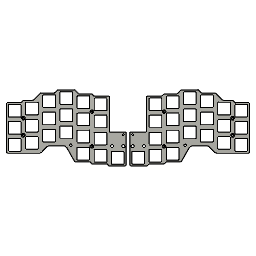
mriya-cnc-top-plate-v.1.01 (Autodesk Fusion 360 design; units mm, degrees)
Autodesk Fusion 360 part; units mm, degrees
sketch "mriya-top-plate" plane through (0, 0, 0) normal (0, 0, 1) x (1, 0, 0)
  line L0 (-96.0213, 15.6719) -> (-89.7787, 21.9145) construction
  line L1 (-21.4858, 1.079) -> (-22.6142, 2.2074) construction
  line L2 (-133.1, 14.7932) -> (-98.1426, 14.7932) construction
  line L3 (-39.0716, 2.7932) -> (-24.0284, 2.7932) construction
  line L4 (-3.6, 0.4932) -> (-20.0716, 0.4932) construction
  line L5 (-59.4741, 6.1094) -> (-67.7517, 20.7608) construction
  line L6 (-40.4858, 3.379) -> (-41.6142, 4.5074) construction
  line L7 (-117.6142, 71.579) -> (-116.4858, 72.7074) construction
  line L8 (-96.0716, 81.2932) -> (-82.2284, 81.2932) construction
  line L9 (-133.1, 70.9932) -> (-119.0284, 70.9932) construction
  line L10 (-87.6574, 22.7932) -> (-71.2344, 22.7932) construction
  line L11 (-43.0284, 5.0932) -> (-57.7328, 5.0932) construction
  line L12 (-77.0716, 84.7932) -> (-59.7284, 84.7932) construction
  line L13 (-53.5716, 80.2932) -> (-40.7284, 80.2932) construction
  line L14 (-20.6, 20.2932) -> (-20.6, 77.9932) construction
  line L15 (-78.4858, 84.2074) -> (-80.8142, 81.879) construction
  line L16 (-58.3142, 84.2074) -> (-54.9858, 80.879) construction
  line L17 (-134.6, 69.4932) -> (-134.6, 16.2932) construction
  line L18 (-38.1858, 78.579) -> (-39.3142, 79.7074) construction
  line L19 (-94.4, 40.3932) -> (-94.4, 27.9932)
  line L20 (-93.6, 41.1932) -> (-81.2, 41.1932)
  line L21 (-93.6, 27.1932) -> (-81.2, 27.1932)
  line L22 (-80.4, 40.3932) -> (-80.4, 27.9932)
  line L23 (-37.4, 56.0932) -> (-37.4, 43.6932)
  line L24 (-36.6, 56.8932) -> (-24.2, 56.8932)
  line L25 (-36.6, 42.8932) -> (-24.2, 42.8932)
  line L26 (-23.4, 56.0932) -> (-23.4, 43.6932)
  line L27 (-56.4, 58.3932) -> (-56.4, 45.9932)
  line L28 (-55.6, 59.1932) -> (-43.2, 59.1932)
  line L29 (-55.6, 45.1932) -> (-43.2, 45.1932)
  line L30 (-42.4, 58.3932) -> (-42.4, 45.9932)
  line L31 (-132.4, 68.0932) -> (-132.4, 55.6932)
  line L32 (-131.6, 68.8932) -> (-119.2, 68.8932)
  line L33 (-131.6, 54.8932) -> (-119.2, 54.8932)
  line L34 (-118.4, 68.0932) -> (-118.4, 55.6932)
  line L35 (-56.4, 39.3932) -> (-56.4, 26.9932)
  line L36 (-55.6, 40.1932) -> (-43.2, 40.1932)
  line L37 (-55.6, 26.1932) -> (-43.2, 26.1932)
  line L38 (-42.4, 39.3932) -> (-42.4, 26.9932)
  line L39 (-37.4, 18.0932) -> (-37.4, 5.6932)
  line L40 (-36.6, 18.8932) -> (-24.2, 18.8932)
  line L41 (-36.6, 4.8932) -> (-24.2, 4.8932)
  line L42 (-23.4, 18.0932) -> (-23.4, 5.6932)
  line L43 (-18.4, 15.7932) -> (-18.4, 3.3932)
  line L44 (-17.6, 16.5932) -> (-5.2, 16.5932)
  line L45 (-17.6, 2.5932) -> (-5.2, 2.5932)
  line L46 (-4.4, 15.7932) -> (-4.4, 3.3932)
  line L47 (-132.4, 49.0932) -> (-132.4, 36.6932)
  line L48 (-131.6, 49.8932) -> (-119.2, 49.8932)
  line L49 (-131.6, 35.8932) -> (-119.2, 35.8932)
  line L50 (-118.4, 49.0932) -> (-118.4, 36.6932)
  line L51 (-113.4, 51.3932) -> (-113.4, 38.9932)
  line L52 (-112.6, 52.1932) -> (-100.2, 52.1932)
  line L53 (-112.6, 38.1932) -> (-100.2, 38.1932)
  line L54 (-99.4, 51.3932) -> (-99.4, 38.9932)
  line L55 (-132.4, 30.0932) -> (-132.4, 17.6932)
  line L56 (-131.6, 30.8932) -> (-119.2, 30.8932)
  line L57 (-131.6, 16.8932) -> (-119.2, 16.8932)
  line L58 (-118.4, 30.0932) -> (-118.4, 17.6932)
  line L59 (-56.4, 20.3932) -> (-56.4, 7.9932)
  line L60 (-55.6, 21.1932) -> (-43.2, 21.1932)
  line L61 (-55.6, 7.1932) -> (-43.2, 7.1932)
  line L62 (-42.4, 20.3932) -> (-42.4, 7.9932)
  line L63 (-75.4, 43.8932) -> (-75.4, 31.4932)
  line L64 (-74.6, 44.6932) -> (-62.2, 44.6932)
  line L65 (-74.6, 30.6932) -> (-62.2, 30.6932)
  line L66 (-61.4, 43.8932) -> (-61.4, 31.4932)
  line L67 (-75.4, 81.8932) -> (-75.4, 69.4932)
  line L68 (-74.6, 82.6932) -> (-62.2, 82.6932)
  line L69 (-74.6, 68.6932) -> (-62.2, 68.6932)
  line L70 (-61.4, 81.8932) -> (-61.4, 69.4932)
  line L71 (-37.4, 37.0932) -> (-37.4, 24.6932)
  line L72 (-36.6, 37.8932) -> (-24.2, 37.8932)
  line L73 (-36.6, 23.8932) -> (-24.2, 23.8932)
  line L74 (-23.4, 37.0932) -> (-23.4, 24.6932)
  line L75 (-113.4, 32.3932) -> (-113.4, 19.9932)
  line L76 (-112.6, 33.1932) -> (-100.2, 33.1932)
  line L77 (-112.6, 19.1932) -> (-100.2, 19.1932)
  line L78 (-99.4, 32.3932) -> (-99.4, 19.9932)
  line L79 (-56.4, 77.3932) -> (-56.4, 64.9932)
  line L80 (-55.6, 78.1932) -> (-43.2, 78.1932)
  line L81 (-55.6, 64.1932) -> (-43.2, 64.1932)
  line L82 (-42.4, 77.3932) -> (-42.4, 64.9932)
  line L83 (-37.4, 75.0932) -> (-37.4, 62.6932)
  line L84 (-36.6, 75.8932) -> (-24.2, 75.8932)
  line L85 (-36.6, 61.8932) -> (-24.2, 61.8932)
  line L86 (-23.4, 75.0932) -> (-23.4, 62.6932)
  line L87 (-113.4, 70.3932) -> (-113.4, 57.9932)
  line L88 (-112.6, 71.1932) -> (-100.2, 71.1932)
  line L89 (-112.6, 57.1932) -> (-100.2, 57.1932)
  line L90 (-99.4, 70.3932) -> (-99.4, 57.9932)
  line L91 (-94.4, 59.3932) -> (-94.4, 46.9932)
  line L92 (-93.6, 60.1932) -> (-81.2, 60.1932)
  line L93 (-93.6, 46.1932) -> (-81.2, 46.1932)
  line L94 (-80.4, 59.3932) -> (-80.4, 46.9932)
  line L95 (-75.4, 62.8932) -> (-75.4, 50.4932)
  line L96 (-74.6, 63.6932) -> (-62.2, 63.6932)
  line L97 (-74.6, 49.6932) -> (-62.2, 49.6932)
  line L98 (-61.4, 62.8932) -> (-61.4, 50.4932)
  line L99 (-94.4, 78.3932) -> (-94.4, 65.9932)
  line L100 (-93.6, 79.1932) -> (-81.2, 79.1932)
  line L101 (-93.6, 65.1932) -> (-81.2, 65.1932)
  line L102 (-80.4, 78.3932) -> (-80.4, 65.9932)
  circle A0 centre (-115.9, 53.5432) radius 1
  circle A1 centre (-115.9, 34.5432) radius 1
  circle A2 centre (-63.3, 23.4932) radius 1.3
  circle A3 centre (-39.9, 22.5432) radius 1
  circle A4 centre (-39.9, 60.5432) radius 1
  arc A5 (-38.1858, 78.579) -> (-36.7716, 77.9932) centre (-36.7716, 79.9932) ccw construction
  arc A6 (-39.3142, 79.7074) -> (-40.7284, 80.2932) centre (-40.7284, 78.2932) ccw construction
  arc A7 (-54.9858, 80.879) -> (-53.5716, 80.2932) centre (-53.5716, 82.2931) ccw construction
  arc A8 (-58.3142, 84.2074) -> (-59.7284, 84.7932) centre (-59.7284, 82.7932) ccw construction
  arc A9 (-77.0716, 84.7932) -> (-78.4858, 84.2074) centre (-77.0716, 82.7933) ccw construction
  arc A10 (-82.2284, 81.2932) -> (-80.8142, 81.879) centre (-82.2284, 83.2932) ccw construction
  arc A11 (-96.0716, 81.2932) -> (-97.4858, 80.7074) centre (-96.0716, 79.2933) ccw construction
  arc A12 (-115.0716, 73.2932) -> (-116.4858, 72.7074) centre (-115.0716, 71.2933) ccw construction
  arc A13 (-119.0284, 70.9932) -> (-117.6142, 71.579) centre (-119.0284, 72.9932) ccw construction
  arc A14 (-133.1, 70.9932) -> (-134.6, 69.4932) centre (-133.1, 69.4932) ccw construction
  arc A15 (-134.6, 16.2932) -> (-133.1, 14.7932) centre (-133.1, 16.2932) ccw construction
  arc A16 (-98.1426, 14.7932) -> (-96.0213, 15.6719) centre (-98.1426, 17.7931) ccw construction
  arc A17 (-87.6574, 22.7932) -> (-89.7787, 21.9145) centre (-87.6573, 19.7931) ccw construction
  arc A18 (-67.7517, 20.7608) -> (-71.2344, 22.7932) centre (-71.2344, 18.793) ccw construction
  arc A19 (-59.4741, 6.1094) -> (-57.7328, 5.0932) centre (-57.7328, 7.0932) ccw construction
  arc A20 (-41.6142, 4.5074) -> (-43.0284, 5.0932) centre (-43.0284, 3.0933) ccw construction
  arc A21 (-40.4858, 3.379) -> (-39.0716, 2.7932) centre (-39.0716, 4.7932) ccw construction
  arc A22 (-22.6142, 2.2074) -> (-24.0284, 2.7932) centre (-24.0284, 0.7933) ccw construction
  arc A23 (-21.4858, 1.079) -> (-20.0716, 0.4932) centre (-20.0716, 2.4932) ccw construction
  arc A24 (-3.6, 0.4932) -> (-2.1, 1.9932) centre (-3.6, 1.9932) ccw construction
  line L103 (-2.1, 1.9932) -> (-2.1, 76.4932) construction
  line L104 (-36.7716, 77.9932) -> (-3.6, 77.9932) construction
  arc A25 (-131.6, 68.8932) -> (-132.4, 68.0932) centre (-131.6, 68.0932) ccw
  arc A26 (-118.4, 68.0932) -> (-119.2, 68.8932) centre (-119.2, 68.0932) ccw
  arc A27 (-119.2, 54.8932) -> (-118.4, 55.6932) centre (-119.2, 55.6932) ccw
  arc A28 (-132.4, 55.6932) -> (-131.6, 54.8932) centre (-131.6, 55.6932) ccw
  arc A29 (-131.6, 49.8932) -> (-132.4, 49.0932) centre (-131.6, 49.0932) ccw
  arc A30 (-118.4, 49.0932) -> (-119.2, 49.8932) centre (-119.2, 49.0932) ccw
  arc A31 (-119.2, 35.8932) -> (-118.4, 36.6932) centre (-119.2, 36.6932) ccw
  arc A32 (-132.4, 36.6932) -> (-131.6, 35.8932) centre (-131.6, 36.6932) ccw
  arc A33 (-131.6, 30.8932) -> (-132.4, 30.0932) centre (-131.6, 30.0932) ccw
  arc A34 (-118.4, 30.0932) -> (-119.2, 30.8932) centre (-119.2, 30.0932) ccw
  arc A35 (-119.2, 16.8932) -> (-118.4, 17.6932) centre (-119.2, 17.6932) ccw
  arc A36 (-132.4, 17.6932) -> (-131.6, 16.8932) centre (-131.6, 17.6932) ccw
  arc A37 (-113.4, 19.9932) -> (-112.6, 19.1932) centre (-112.6, 19.9932) ccw
  arc A38 (-100.2, 19.1932) -> (-99.4, 19.9932) centre (-100.2, 19.9932) ccw
  arc A39 (-99.4, 32.3932) -> (-100.2, 33.1932) centre (-100.2, 32.3932) ccw
  arc A40 (-112.6, 33.1932) -> (-113.4, 32.3932) centre (-112.6, 32.3932) ccw
  arc A41 (-100.2, 38.1932) -> (-99.4, 38.9932) centre (-100.2, 38.9932) ccw
  arc A42 (-113.4, 38.9932) -> (-112.6, 38.1932) centre (-112.6, 38.9932) ccw
  arc A43 (-112.6, 52.1932) -> (-113.4, 51.3932) centre (-112.6, 51.3932) ccw
  arc A44 (-99.4, 51.3932) -> (-100.2, 52.1932) centre (-100.2, 51.3932) ccw
  arc A45 (-113.4, 57.9932) -> (-112.6, 57.1932) centre (-112.6, 57.9932) ccw
  arc A46 (-100.2, 57.1932) -> (-99.4, 57.9932) centre (-100.2, 57.9932) ccw
  arc A47 (-99.4, 70.3932) -> (-100.2, 71.1932) centre (-100.2, 70.3932) ccw
  arc A48 (-112.6, 71.1932) -> (-113.4, 70.3932) centre (-112.6, 70.3932) ccw
  arc A49 (-93.6, 79.1932) -> (-94.4, 78.3932) centre (-93.6, 78.3932) ccw
  arc A50 (-80.4, 78.3932) -> (-81.2, 79.1932) centre (-81.2, 78.3932) ccw
  arc A51 (-81.2, 65.1932) -> (-80.4, 65.9932) centre (-81.2, 65.9932) ccw
  arc A52 (-94.4, 65.9932) -> (-93.6, 65.1932) centre (-93.6, 65.9932) ccw
  arc A53 (-93.6, 60.1932) -> (-94.4, 59.3932) centre (-93.6, 59.3932) ccw
  arc A54 (-80.4, 59.3932) -> (-81.2, 60.1932) centre (-81.2, 59.3932) ccw
  arc A55 (-81.2, 46.1932) -> (-80.4, 46.9932) centre (-81.2, 46.9932) ccw
  arc A56 (-94.4, 46.9932) -> (-93.6, 46.1932) centre (-93.6, 46.9932) ccw
  arc A57 (-93.6, 41.1932) -> (-94.4, 40.3932) centre (-93.6, 40.3932) ccw
  arc A58 (-94.4, 27.9932) -> (-93.6, 27.1932) centre (-93.6, 27.9932) ccw
  arc A59 (-81.2, 27.1932) -> (-80.4, 27.9932) centre (-81.2, 27.9932) ccw
  arc A60 (-80.4, 40.3932) -> (-81.2, 41.1932) centre (-81.2, 40.3932) ccw
  arc A61 (-75.4, 31.4932) -> (-74.6, 30.6932) centre (-74.6, 31.4932) ccw
  arc A62 (-74.6, 44.6932) -> (-75.4, 43.8932) centre (-74.6, 43.8932) ccw
  arc A63 (-61.4, 43.8932) -> (-62.2, 44.6932) centre (-62.2, 43.8932) ccw
  arc A64 (-62.2, 30.6932) -> (-61.4, 31.4932) centre (-62.2, 31.4932) ccw
  arc A65 (-62.2, 49.6932) -> (-61.4, 50.4932) centre (-62.2, 50.4932) ccw
  arc A66 (-75.4, 50.4932) -> (-74.6, 49.6932) centre (-74.6, 50.4932) ccw
  arc A67 (-74.6, 63.6932) -> (-75.4, 62.8932) centre (-74.6, 62.8932) ccw
  arc A68 (-61.4, 62.8932) -> (-62.2, 63.6932) centre (-62.2, 62.8932) ccw
  arc A69 (-62.2, 68.6932) -> (-61.4, 69.4932) centre (-62.2, 69.4932) ccw
  arc A70 (-75.4, 69.4932) -> (-74.6, 68.6932) centre (-74.6, 69.4932) ccw
  arc A71 (-74.6, 82.6932) -> (-75.4, 81.8932) centre (-74.6, 81.8932) ccw
  arc A72 (-61.4, 81.8932) -> (-62.2, 82.6932) centre (-62.2, 81.8932) ccw
  arc A73 (-55.6, 78.1932) -> (-56.4, 77.3932) centre (-55.6, 77.3932) ccw
  arc A74 (-56.4, 64.9932) -> (-55.6, 64.1932) centre (-55.6, 64.9932) ccw
  arc A75 (-43.2, 64.1932) -> (-42.4, 64.9932) centre (-43.2, 64.9932) ccw
  arc A76 (-42.4, 77.3932) -> (-43.2, 78.1932) centre (-43.2, 77.3932) ccw
  arc A77 (-42.4, 58.3932) -> (-43.2, 59.1932) centre (-43.2, 58.3932) ccw
  arc A78 (-55.6, 59.1932) -> (-56.4, 58.3932) centre (-55.6, 58.3932) ccw
  arc A79 (-56.4, 45.9932) -> (-55.6, 45.1932) centre (-55.6, 45.9932) ccw
  arc A80 (-43.2, 45.1932) -> (-42.4, 45.9932) centre (-43.2, 45.9932) ccw
  arc A81 (-42.4, 39.3932) -> (-43.2, 40.1932) centre (-43.2, 39.3932) ccw
  arc A82 (-55.6, 40.1932) -> (-56.4, 39.3932) centre (-55.6, 39.3932) ccw
  arc A83 (-56.4, 26.9932) -> (-55.6, 26.1932) centre (-55.6, 26.9932) ccw
  arc A84 (-43.2, 26.1932) -> (-42.4, 26.9932) centre (-43.2, 26.9932) ccw
  arc A85 (-42.4, 20.3932) -> (-43.2, 21.1932) centre (-43.2, 20.3932) ccw
  arc A86 (-55.6, 21.1932) -> (-56.4, 20.3932) centre (-55.6, 20.3932) ccw
  arc A87 (-56.4, 7.9932) -> (-55.6, 7.1932) centre (-55.6, 7.9932) ccw
  arc A88 (-43.2, 7.1932) -> (-42.4, 7.9932) centre (-43.2, 7.9932) ccw
  arc A89 (-37.4, 5.6932) -> (-36.6, 4.8932) centre (-36.6, 5.6932) ccw
  arc A90 (-24.2, 4.8932) -> (-23.4, 5.6932) centre (-24.2, 5.6932) ccw
  arc A91 (-23.4, 18.0932) -> (-24.2, 18.8932) centre (-24.2, 18.0932) ccw
  arc A92 (-36.6, 18.8932) -> (-37.4, 18.0932) centre (-36.6, 18.0932) ccw
  arc A93 (-18.4, 3.3932) -> (-17.6, 2.5932) centre (-17.6, 3.3932) ccw
  arc A94 (-5.2, 2.5932) -> (-4.4, 3.3932) centre (-5.2, 3.3932) ccw
  arc A95 (-4.4, 15.7932) -> (-5.2, 16.5932) centre (-5.2, 15.7932) ccw
  arc A96 (-17.6, 16.5932) -> (-18.4, 15.7932) centre (-17.6, 15.7932) ccw
  arc A97 (-24.2, 23.8932) -> (-23.4, 24.6932) centre (-24.2, 24.6932) ccw
  arc A98 (-37.4, 24.6932) -> (-36.6, 23.8932) centre (-36.6, 24.6932) ccw
  arc A99 (-36.6, 37.8932) -> (-37.4, 37.0932) centre (-36.6, 37.0932) ccw
  arc A100 (-23.4, 37.0932) -> (-24.2, 37.8932) centre (-24.2, 37.0932) ccw
  arc A101 (-24.2, 42.8932) -> (-23.4, 43.6932) centre (-24.2, 43.6932) ccw
  arc A102 (-37.4, 43.6932) -> (-36.6, 42.8932) centre (-36.6, 43.6932) ccw
  arc A103 (-36.6, 56.8932) -> (-37.4, 56.0932) centre (-36.6, 56.0932) ccw
  arc A104 (-23.4, 56.0932) -> (-24.2, 56.8932) centre (-24.2, 56.0932) ccw
  arc A105 (-24.2, 61.8932) -> (-23.4, 62.6932) centre (-24.2, 62.6932) ccw
  arc A106 (-37.4, 62.6932) -> (-36.6, 61.8932) centre (-36.6, 62.6932) ccw
  arc A107 (-36.6, 75.8932) -> (-37.4, 75.0932) centre (-36.6, 75.0932) ccw
  arc A108 (-23.4, 75.0932) -> (-24.2, 75.8932) centre (-24.2, 75.0932) ccw
  circle A109 centre (-115.9, 53.5432) radius 2
  circle A110 centre (-115.9, 34.5432) radius 2
  circle A111 centre (-39.9, 22.5432) radius 2
  circle A112 centre (-39.9, 60.5432) radius 2
  line L105 (-104.0213, 74.1719) -> (-97.4858, 80.7074) construction
  line L106 (-106.1426, 73.2932) -> (-115.0716, 73.2932) construction
  arc A113 (-106.1426, 73.2932) -> (-104.0213, 74.1719) centre (-106.1426, 76.2932) ccw construction
  circle A114 centre (-5.1, 22.4932) radius 1.7
  circle A115 centre (-17.6, 22.4932) radius 1.7
  line L107 (-19.7, 38.1932) -> (-2.85, 38.1932)
  line L108 (-20.7, 39.1932) -> (-20.7, 77.2432)
  line L109 (-36.7716, 78.0432) -> (-21.5, 78.0432)
  arc A116 (-38.1504, 78.6144) -> (-36.7716, 78.0432) centre (-36.7716, 79.9932) ccw
  line L110 (-38.1504, 78.6144) -> (-39.2788, 79.7428)
  arc A117 (-39.2788, 79.7428) -> (-40.7284, 80.3432) centre (-40.7284, 78.2932) ccw
  line L111 (-53.5716, 80.3432) -> (-40.7284, 80.3432)
  arc A118 (-54.9504, 80.9144) -> (-53.5716, 80.3432) centre (-53.5716, 82.2931) ccw
  line L112 (-58.2788, 84.2428) -> (-54.9504, 80.9144)
  arc A119 (-58.2788, 84.2428) -> (-59.7284, 84.8432) centre (-59.7284, 82.7932) ccw
  line L113 (-77.0716, 84.8432) -> (-59.7284, 84.8432)
  arc A120 (-77.0716, 84.8432) -> (-78.5212, 84.2428) centre (-77.0716, 82.7933) ccw
  line L114 (-78.5212, 84.2428) -> (-80.8496, 81.9144)
  arc A121 (-82.2284, 81.3432) -> (-80.8496, 81.9144) centre (-82.2284, 83.2932) ccw
  line L115 (-96.0716, 81.3432) -> (-82.2284, 81.3432)
  arc A122 (-96.0716, 81.3432) -> (-97.5211, 80.7428) centre (-96.0716, 79.2933) ccw
  line L116 (-104.0567, 74.2072) -> (-97.5211, 80.7428)
  arc A123 (-106.1426, 73.3432) -> (-104.0567, 74.2072) centre (-106.1426, 76.2932) ccw
  line L117 (-106.1426, 73.3432) -> (-115.0716, 73.3432)
  arc A124 (-115.0716, 73.3432) -> (-116.5212, 72.7428) centre (-115.0716, 71.2933) ccw
  line L118 (-117.6496, 71.6144) -> (-116.5212, 72.7428)
  arc A125 (-119.0284, 71.0432) -> (-117.6496, 71.6144) centre (-119.0284, 72.9932) ccw
  line L119 (-133.1, 71.0432) -> (-119.0284, 71.0432)
  arc A126 (-133.1, 71.0432) -> (-134.65, 69.4932) centre (-133.1, 69.4932) ccw
  line L120 (-134.65, 69.4932) -> (-134.65, 16.2932)
  arc A127 (-134.65, 16.2932) -> (-133.1, 14.7432) centre (-133.1, 16.2932) ccw
  line L121 (-133.1, 14.7432) -> (-98.1426, 14.7432)
  arc A128 (-98.1426, 14.7432) -> (-95.9859, 15.6365) centre (-98.1426, 17.7931) ccw
  line L122 (-95.9859, 15.6365) -> (-89.7433, 21.8791)
  arc A129 (-87.6574, 22.7432) -> (-89.7433, 21.8791) centre (-87.6573, 19.7931) ccw
  line L123 (-87.6574, 22.7432) -> (-71.2344, 22.7432)
  arc A130 (-67.7952, 20.7362) -> (-71.2344, 22.7432) centre (-71.2344, 18.793) ccw
  line L124 (-59.5176, 6.0848) -> (-67.7952, 20.7362)
  arc A131 (-59.5176, 6.0848) -> (-57.7328, 5.0432) centre (-57.7328, 7.0932) ccw
  line L125 (-43.0284, 5.0432) -> (-57.7328, 5.0432)
  arc A132 (-41.6496, 4.472) -> (-43.0284, 5.0432) centre (-43.0284, 3.0933) ccw
  line L126 (-40.5212, 3.3436) -> (-41.6496, 4.472)
  arc A133 (-40.5212, 3.3436) -> (-39.0716, 2.7432) centre (-39.0716, 4.7932) ccw
  line L127 (-39.0716, 2.7432) -> (-24.0284, 2.7432)
  arc A134 (-22.6496, 2.172) -> (-24.0284, 2.7432) centre (-24.0284, 0.7933) ccw
  line L128 (-21.5212, 1.0436) -> (-22.6496, 2.172)
  arc A135 (-21.5212, 1.0436) -> (-20.0716, 0.4432) centre (-20.0716, 2.4932) ccw
  line L129 (-3.6, 0.4432) -> (-20.0716, 0.4432)
  arc A136 (-3.6, 0.4432) -> (-2.05, 1.9932) centre (-3.6, 1.9932) ccw
  line L130 (-2.05, 1.9932) -> (-2.05, 37.3932)
  line L131 (-19.8, 19.4932) -> (-2.1, 19.4932) construction
  arc A137 (-20.7, 77.2432) -> (-21.5, 78.0432) centre (-21.5, 77.2432) ccw
  arc A138 (-2.1, 76.4932) -> (-3.6, 77.9932) centre (-3.6, 76.4932) ccw construction
  arc A139 (-20.6, 20.2932) -> (-19.8, 19.4932) centre (-19.8, 20.2932) ccw construction
  circle A140 centre (-17.6, 22.4932) radius 1 construction
  circle A141 centre (-5.1, 22.4932) radius 1 construction
  line L132 (-12.7, 24.1932) -> (-10.1, 24.1932) construction
  line L133 (-10.1, 20.7932) -> (-12.7, 20.7932) construction
  arc A142 (-10.1, 20.7932) -> (-10.1, 24.1932) centre (-10.1, 22.4932) ccw construction
  arc A143 (-12.7, 24.1932) -> (-12.7, 20.7932) centre (-12.7, 22.4932) ccw construction
  arc A144 (-20.7, 39.1932) -> (-19.7, 38.1932) centre (-19.7, 39.1932) ccw
  arc A145 (-2.05, 37.3932) -> (-2.85, 38.1932) centre (-2.85, 37.3932) ccw
  circle A146 centre (-5.1, 35.1932) radius 1
  dimension "d1" = 2
  dimension "d2" = 2
  dimension "d3" = 2.6
  dimension "d4" = 2
  dimension "d5" = 2
  dimension "d17" = 4
  dimension "d18" = 4
  dimension "d19" = 4
  dimension "d20" = 4
  dimension "d33" = 3.4
  dimension "d35" = 3.4
  dimension "d358" = 2
  constraint tangent L18 A5
  constraint tangent L18 A6
  constraint tangent L13 A7
  constraint tangent L16 A8
  constraint tangent L12 A9
  constraint tangent L15 A10
  constraint tangent L8 A11
  constraint tangent L7 A13
  constraint tangent L9 A14
  constraint tangent L17 A15
  constraint tangent L2 A16
  constraint tangent L0 A17
  constraint tangent L10 A18
  constraint tangent L5 A19
  constraint tangent L11 A20
  constraint tangent L6 A21
  constraint tangent L3 A22
  constraint tangent L1 A23
  constraint tangent L4 A24
  constraint tangent A24 L103
  constraint perpendicular L103 L104
  constraint perpendicular L14 L104
  constraint perpendicular L103 L131
  constraint tangent L31 A25
  constraint tangent L32 A26
  constraint tangent L34 A27
  constraint tangent L33 A28
  constraint tangent L48 A29
  constraint tangent L48 A30
  constraint tangent L50 A31
  constraint tangent L49 A32
  constraint tangent L56 A33
  constraint tangent L56 A34
  constraint tangent L58 A35
  constraint tangent L57 A36
  constraint tangent L75 A37
  constraint tangent L77 A38
  constraint tangent L78 A39
  constraint tangent L76 A40
  constraint tangent L53 A41
  constraint tangent L53 A42
  constraint tangent L51 A43
  constraint tangent L52 A44
  constraint tangent L89 A45
  constraint tangent L89 A46
  constraint tangent L90 A46
  constraint tangent L90 A47
  constraint tangent L88 A48
  constraint tangent L99 A49
  constraint tangent L100 A50
  constraint tangent L102 A51
  constraint tangent L101 A52
  constraint tangent L92 A53
  constraint tangent L92 A54
  constraint tangent L94 A55
  constraint tangent L93 A56
  constraint tangent L20 A57
  constraint tangent L19 A58
  constraint tangent L21 A58
  constraint tangent L21 A59
  constraint tangent L22 A60
  constraint tangent L63 A61
  constraint tangent L65 A61
  constraint tangent L63 A62
  constraint tangent L64 A63
  constraint tangent L66 A64
  constraint tangent L97 A65
  constraint tangent L97 A66
  constraint tangent L95 A67
  constraint tangent L96 A68
  constraint tangent L69 A69
  constraint tangent L69 A70
  constraint tangent L67 A71
  constraint tangent L68 A72
  constraint tangent L79 A73
  constraint tangent L79 A74
  constraint tangent L81 A74
  constraint tangent L81 A75
  constraint tangent L82 A75
  constraint tangent L82 A76
  constraint tangent L80 A76
  constraint tangent L28 A77
  constraint tangent L28 A78
  constraint tangent L27 A79
  constraint tangent L29 A80
  constraint tangent L36 A81
  constraint tangent L36 A82
  constraint tangent L35 A82
  constraint tangent L35 A83
  constraint tangent L37 A83
  constraint tangent L37 A84
  constraint tangent L38 A84
  constraint tangent L60 A85
  constraint tangent L60 A86
  constraint tangent L59 A86
  constraint tangent L59 A87
  constraint tangent L61 A88
  constraint tangent L39 A89
  constraint tangent L41 A90
  constraint tangent L42 A91
  constraint tangent L40 A91
  constraint tangent L40 A92
  constraint tangent L39 A92
  constraint tangent L43 A93
  constraint tangent L45 A93
  constraint tangent L45 A94
  constraint tangent L46 A94
  constraint tangent L46 A95
  constraint tangent L44 A95
  constraint tangent L44 A96
  constraint tangent L43 A96
  constraint tangent L73 A97
  constraint tangent L74 A97
  constraint tangent L73 A98
  constraint tangent L71 A99
  constraint tangent L72 A100
  constraint tangent L25 A101
  constraint tangent L26 A101
  constraint tangent L25 A102
  constraint tangent L23 A103
  constraint tangent L24 A104
  constraint tangent L85 A105
  constraint tangent L86 A105
  constraint tangent L85 A106
  constraint tangent L83 A107
  constraint tangent L84 A108
  constraint concentric A0 A109
  constraint concentric A1 A110
  constraint concentric A3 A111
  constraint concentric A4 A112
  constraint tangent A11 L105
  constraint tangent A12 L106
  constraint tangent L105 A113
  constraint tangent L106 A113
  constraint horizontal L131
  constraint concentric A5 A116
  constraint concentric A6 A117
  constraint concentric A7 A118
  constraint concentric A8 A119
  constraint concentric A9 A120
  constraint concentric A10 A121
  constraint concentric A11 A122
  constraint concentric A113 A123
  constraint concentric A12 A124
  constraint concentric A13 A125
  constraint concentric A14 A126
  constraint concentric A15 A127
  constraint concentric A16 A128
  constraint concentric A17 A129
  constraint concentric A18 A130
  constraint concentric A19 A131
  constraint concentric A20 A132
  constraint concentric A21 A133
  constraint concentric A22 A134
  constraint concentric A23 A135
  constraint concentric A24 A136
  constraint tangent L113 A120
  constraint tangent A116 L110
  constraint tangent L110 A117
  constraint tangent A123 L117
  constraint tangent A127 L121
  constraint tangent L115 A122
  constraint tangent L121 A128
  constraint tangent L119 A126
  constraint tangent L117 A124
  constraint tangent A136 L130
  constraint tangent A126 L120
  constraint tangent L120 A127
  constraint tangent L123 A130
  constraint tangent L125 A132
  constraint tangent L127 A134
  constraint tangent L129 A136
  constraint tangent L108 A137
  constraint tangent L109 A137
  constraint tangent L104 A138
  constraint tangent L103 A138
  constraint coincident L104 L14.end
  constraint tangent L131 A139
  constraint tangent L14 A139
  constraint concentric A115 A140
  constraint concentric A114 A141
  constraint tangent L133 A143
  constraint coincident L133 A142.start
  constraint tangent L108 A144
  constraint tangent L107 A144
  constraint tangent L107 A145
  constraint tangent L130 A145
  measures "d1" diameter of A0
  measures "d2" diameter of A1
  measures "d3" diameter of A2
  measures "d4" diameter of A3
  measures "d5" diameter of A4
  measures "d17" diameter of A109
  measures "d18" diameter of A110
  measures "d19" diameter of A111
  measures "d20" diameter of A112
  measures "d33" diameter of A114
  measures "d35" diameter of A115
  measures "d358" diameter of A146
extrude "Extrude1" add sketch "mriya-top-plate" along normal blind 1.5 contours L107 L108 L109 A116 L110 A117 L111 A118 L112 A119 L113 A120 L114 A121 L115 A122 L116 A123 L117 A124 L118 A125 L119 A126 L120 A127 L121 A128 L122 A129 L123 A130 L124 A131 L125 A132 L126 A133 L127 A134 L128 A135 L129 A136 L130 A137 A144 A145 makes body 1
extrude "Extrude25" add sketch "mriya-top-plate" along normal blind 0.7 contours A109 | A110 | A111 | A112 bodies 1
mirror "Mirror1" about plane through (0, 0, 0) normal (1, 0, 0) of bodies 1 makes body 2
named bodies: "Left", "Right"
